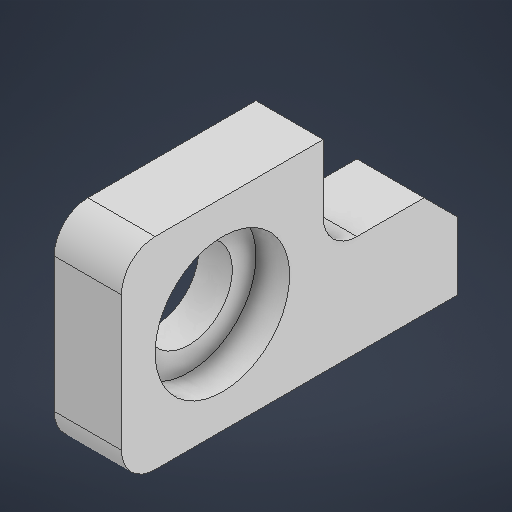
# Autodesk Inventor part: Part4
Saved by Autodesk Inventor 2026 (Build 300175050, 175E)
## iProperties
Created: 2026-03-19
Part Number: Part4
Material: Generic
Document SubType Name: Modeling
Designer: Administrator
Density: 1 g/cm^3
Appearance: Default
Author: Administrator
Autodesk Inventor part; units mm, degrees
ref_plane "YZ Plane" through (0, 0, 0) normal (1, 0, 0) x (0, 1, 0)
ref_plane "XZ Plane" through (0, 0, 0) normal (0, 1, 0) x (-1, 0, 0)
ref_plane "XY Plane" through (0, 0, 0) normal (0, 0, 1) x (1, 0, 0)
sketch "Sketch1" plane through (0, 0, 0) normal (1, 0, 0) x (0, 1, 0)
  line L0 (0, 0) -> (0, -100)
  line L1 (0, -100) -> (30, -100)
  line L2 (30, -100) -> (30, -60)
  line L3 (30, -60) -> (60, -60)
  line L4 (60, -60) -> (60, 0)
  line L5 (60, 0) -> (0, 0)
  dimension "d0" = 60
  dimension "d1" = 30
  dimension "d2" = 30
  dimension "d3" = 40
  dimension "d4" = 60
  dimension "d5" = 100
  constraints: 12 end point, 5 perpendicular, 1 vertical
  measures "d0" distance of L3.end L4.end
  measures "d1" distance of L2.end L3.end
  measures "d2" distance of L0.end L1.end
  measures "d3" distance of L1.end L2.end
  measures "d4" distance of L4.end L0.start
  measures "d5" distance of L0.start L0.end
extrude "Extrusion1" add sketch "Sketch1" along normal blind 20
chamfer "Chamfer1" distance 10 angle 45 1 edges at (10, 30, -100)
fillet "Fillet1" radius 10 1 edges at (10, 0, 0)
fillet "Fillet2" radius 10 1 edges at (10, 30, -60)
fillet "Fillet3" radius 10 1 edges at (10, 60, 0)
sketch "Sketch2" plane through (20, 0, 0) normal (1, 0, 0) x (0, 0, -1)
  circle A0 centre (30, 30) radius 20
  line L0 (10, 0) -> (100, 0) projected
  line L1 (0, 50) -> (0, 10) projected
  point P0 (0, 0)
  dimension "d14" = 30
  dimension "d15" = 30
  dimension "d16" = 40
  constraints: 1 centre point
  measures "d14" distance from line of A0.centre L0
  measures "d15" distance from line of A0.centre L1
  measures "d16" diameter of A0
extrude "Extrusion2" cut sketch "Sketch2" against normal blind 10
sketch "Sketch3" plane through (10, 30, -30) normal (1, 0, 0) x (0, 0, -1)
  circle A0 centre (0, 0) radius 12.9798
  line L0 (-20, -30) -> (70, -30) projected
  line L1 (-30, 20) -> (-30, -20) projected
  point P0 (-30, -30)
  dimension "d19" = 30
  dimension "d20" = 30
  constraints: 1 centre point
  measures "d19" distance from line of A0.centre L0
  measures "d20" distance from line of A0.centre L1
extrude "Extrusion3" cut sketch "Sketch3" against normal blind 20
body "Solid1"
